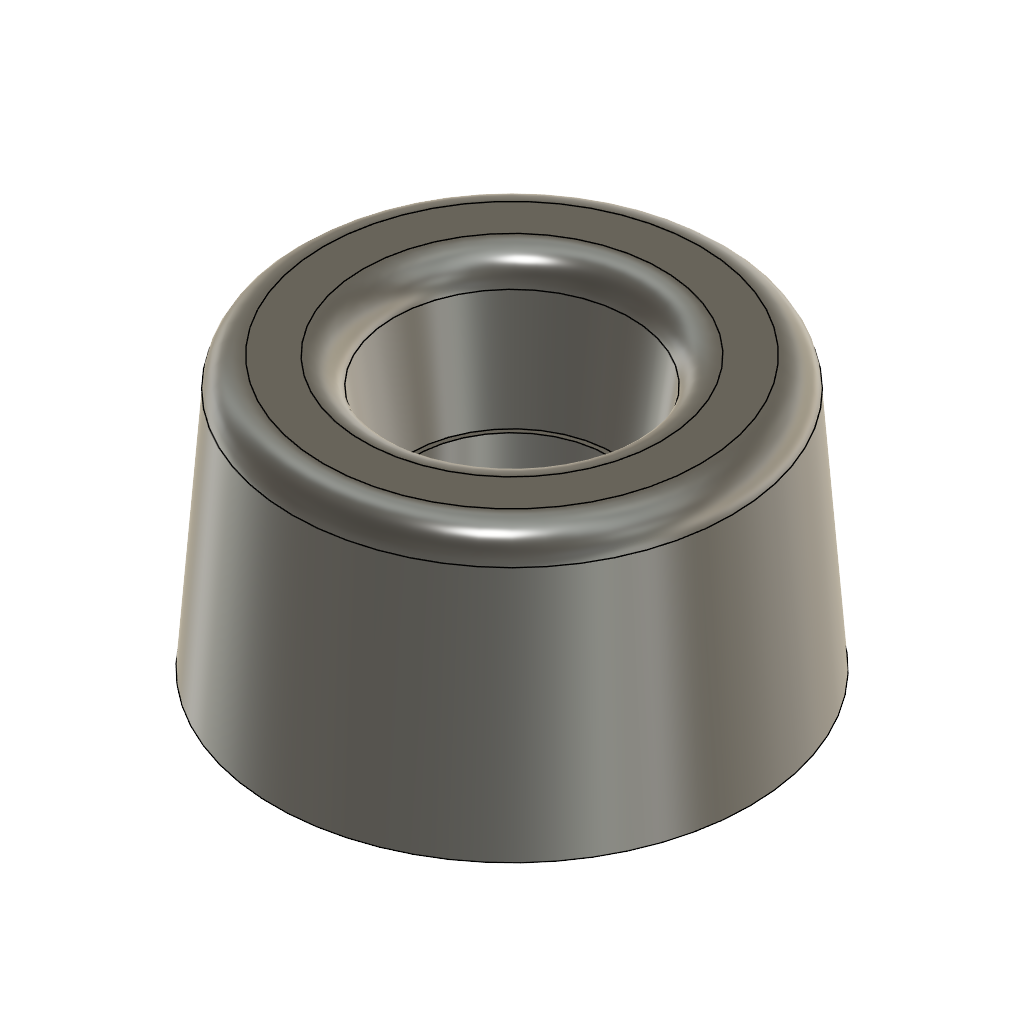
Rubber Footsie (Autodesk Fusion 360 design; units mm, degrees)
Autodesk Fusion 360 part; units mm, degrees
sketch "Sketch1" plane through (0, 0, 0) normal (0, 0, 1) x (1, 0, 0)
  circle A0 centre (0, 0) radius 17.5
  dimension "d1" = 35
  constraint coincident A0.centre origin
  measures "d1" diameter of A0
ref_plane "WorkPlane1" through (0, 0, 20) normal (0, 0, 1) x (1, 0, 0)
sketch "Sketch2" plane through (0, 0, 20) normal (0, 0, 1) x (1, 0, 0)
  circle A0 centre (0, 0) radius 16
  dimension "d3" = 32
  constraint coincident A0.centre origin
  measures "d3" diameter of A0
loft "Loft1" add profiles "Sketch1", "Sketch2" section 1 section 2
ref_plane "WorkPlane2" through (0, 0, 10) normal (0, 0, 1) x (1, 0, 0)
sketch "Sketch3" plane through (0, 0, 10) normal (0, 0, 1) x (1, 0, 0)
  circle A0 centre (0, 0) radius 7.5
  dimension "d5" = 15
  constraint coincident A0.centre origin
  measures "d5" diameter of A0
sketch "Sketch4" plane through (0, 0, 20) normal (0, 0, 1) x (-1, 0, 0)
  circle A0 centre (0, 0) radius 16
  circle A1 centre (0, 0) radius 9
  dimension "d6" = 18
  constraint coincident A0.centre A1.centre
  measures "d6" diameter of A1
loft "Loft2" cut profiles "Sketch3", "Sketch4" section 1 section 2 contours A1
fillet "Fillet1" radius 2.3 2 edges at (8.3909, -3.2545, 20) (-14.9172, 5.7858, 20)
sketch "Sketch5" plane through (0, 0, 10) normal (0, 0, 1) x (-1, 0, 0)
  circle A0 centre (0, 0) radius 7.5
  circle A1 centre (0, 0) radius 4.575
  dimension "d9" = 9.15
  constraint coincident A0.centre A1.centre
  measures "d9" diameter of A1
extrude "Extrude1" cut sketch "Sketch5" against normal blind 10 contours A1
sketch "Sketch6" plane through (0, 0, 10) normal (0, 0, 1) x (-1, 0, 0)
  circle A0 centre (0, 0) radius 4.575
  circle A1 centre (0, 0) radius 7.5
  circle A2 centre (0, 0) radius 7.15
  dimension "d12" = 14.3
  constraint coincident A0.centre A1.centre
  measures "d12" diameter of A2
extrude "Extrude2" cut sketch "Sketch6" against normal blind 5 contours A2
equation "d4 = -20 mm + 10 mm"
